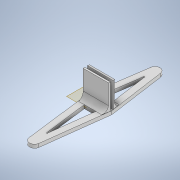
# Autodesk Inventor part: support
Saved by Autodesk Inventor 2020 (Build 240168000, 168)
## iProperties
Created: 2020-07-18
Part Number: support
Material: Generic
Document SubType Name: Modeling
Designer: gerac
Density: 1 g/cm^3
Appearance: Default
Author: gerac
Autodesk Inventor part; units mm, degrees
ref_plane "YZ Plane" through (0, 0, 0) normal (1, 0, 0) x (0, 1, 0)
ref_plane "XZ Plane" through (0, 0, 0) normal (0, 1, 0) x (-1, 0, 0)
ref_plane "XY Plane" through (0, 0, 0) normal (0, 0, 1) x (1, 0, 0)
sketch "Sketch1" plane through (0, 0, 0) normal (0, 1, 0) x (-1, 0, 0)
  line L0 (0, 0) -> (-30, 0)
  line L1 (-30, 0) -> (-20, -70)
  line L2 (-20, -70) -> (-10, -70)
  line L3 (-10, -70) -> (0, 0)
  line L4 (-30, 0) -> (-20, 80)
  line L5 (-20, 80) -> (-10, 80)
  line L6 (-10, 80) -> (0, 0)
  line L7 (-21.6955, 10) -> (-8.3045, 10)
  line L8 (-8.3045, 10) -> (-15, 63.5642)
  line L9 (-15, 63.5642) -> (-21.6955, 10)
  line L10 (-21.5004, -10) -> (-8.4996, -10)
  line L11 (-8.4996, -10) -> (-15, -55.5025)
  line L12 (-15, -55.5025) -> (-21.5004, -10)
  dimension "d15" = 80
  dimension "d16" = 70
  dimension "d17" = 10
  dimension "d18" = 10
  dimension "d19" = 30
  dimension "d20" = 10
  dimension "d21" = 10
  dimension "d40" = 10
  dimension "d41" = 10
  dimension "d42" = 7
  dimension "d43" = 7
  dimension "d45" = 7
  dimension "d46" = 7
  constraints: 29 end point, 6 parallel, 3 horizontal
  measures "d15" distance between parallel lines of L0 L5
  measures "d16" distance between parallel lines of L2 L0
  measures "d17" horizontal distance of L1.end L0.end
  measures "d18" horizontal distance of L2.end L0.start
  measures "d19" distance of L0.start L0.end
  measures "d20" horizontal distance of L0.start L5.end
  measures "d21" horizontal distance of L4.end L0.end
  measures "d40" distance between parallel lines of L0 L7
  measures "d41" distance between parallel lines of L10 L0
  measures "d42" distance between parallel lines of L1 L12
  measures "d43" distance between parallel lines of L11 L3
  measures "d45" distance between parallel lines of L4 L9
  measures "d46" distance between parallel lines of L8 L6
ref_plane "Work Plane2" through (0, 3, 0) normal (0, 1, 0) x (1, 0, 0)
sketch "Sketch3" plane through (0, 3, 0) normal (0, 1, 0) x (1, 0, 0)
  line L0 (30, 0) -> (20, 50) projected
  line L1 (20, -60) -> (30, 0) projected
  line L2 (0, 0) -> (10, -60) projected
  line L3 (10, 50) -> (0, 0) projected
  line L4 (29.1194, -1.55) -> (0.2583, -1.55)
  line L5 (0.5917, -3.55) -> (0.2583, -1.55)
  line L6 (0.5917, -3.55) -> (29.4083, -3.55)
  line L7 (29.69, 1.55) -> (29.29, 3.55)
  line L8 (29.29, 3.55) -> (0.71, 3.55)
  line L9 (0.71, 3.55) -> (0.31, 1.55)
  line L10 (0.31, 1.55) -> (29.69, 1.55)
  line L11 (30, 0) -> (0, 0)
  line L12 (29.4083, -3.55) -> (29.7417, -1.55)
  line L13 (29.1194, -1.55) -> (29.7417, -1.55)
  dimension "d26" = 1.55
  dimension "d27" = 1.55
  dimension "d28" = 2
  dimension "d29" = 2
  constraints: 20 end point, 8 point on line, 4 parallel, 2 horizontal
  measures "d26" distance between parallel lines of L11 L4
  measures "d27" distance between parallel lines of L10 L11
  measures "d28" distance between parallel lines of L10 L8
  measures "d29" distance between parallel lines of L6 L4
extrude "Extrusion5" add sketch "Sketch1" along normal blind 4
fillet "Fillet3" radius 5.75 4 edges at (20, 2, 80) (10, 2, 80) (20, 2, -70) (10, 2, -70)
fillet "Fillet4" radius 0.5 2 edges at (15, 2, 63.5642) (15, 2, -55.5025)
extrude "Extrusion7" add sketch "Sketch3" along normal blind 30 contours L10 L3 L8 L0 | L1 L6 L2 L4 L13
fillet "Fillet5" radius 6.45 2 edges at (15, 4, -3.55) (15, 4, 3.55)
equation "\"d18\" = d17"
equation "\"d20\" = d17"
equation "\"d21\" = d17"
equation "\"d43\" = d42"
equation "\"d45\" = d42"
equation "\"d46\" = d42"
equation "\"d27\" = d26"
equation "\"d29\" = d28"
body "Solid2"
